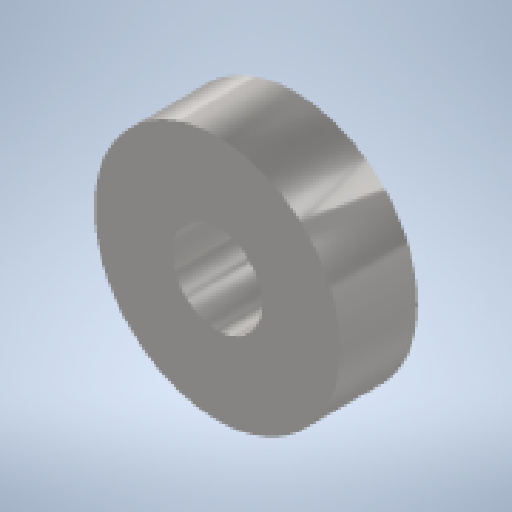
# Autodesk Inventor part: Metal bearing
Saved by Autodesk Inventor 2025.3 (Build 293356000, 356)
## iProperties
Created: 2025-08-19
Part Number: Metal bearing
Material: Stainless Steel
Document SubType Name: Modeling
Designer: sniel
Density: 8 g/cm^3
Appearance: Semi-Polished
Author: sniel
Autodesk Inventor part; units mm, degrees
ref_plane "YZ Plane" through (0, 0, 0) normal (1, 0, 0) x (0, 1, 0)
ref_plane "XZ Plane" through (0, 0, 0) normal (0, 1, 0) x (-1, 0, 0)
ref_plane "XY Plane" through (0, 0, 0) normal (0, 0, 1) x (1, 0, 0)
sketch "Sketch1" plane through (0, 0, 0) normal (0, 0, 1) x (1, 0, 0)
  circle A0 centre (32.4852, 19.5525) radius 11.1
  point P0 (0, 0)
  constraints: 1 centre point
extrude "Extrusion1" add sketch "Sketch1" along normal blind 7
sketch "Sketch7" plane through (32.4852, 19.5525, 7) normal (0, 0, 1) x (1, 0, 0)
  circle A0 centre (0, 0) radius 4.05
  circle A1 centre (0, 0) radius 11.1
  point P0 (-32.4852, -19.5525)
  constraints: 2 centre point
extrude "Extrusion7" cut sketch "Sketch7" against normal up to surface (7 mm away) contours A0
sketch "Sketch8" plane through (32.4852, 19.5525, 7) normal (0, 0, 1) x (1, 0, 0)
  circle A0 centre (0, 0) radius 4.05 projected
  line L0 (4.05, 0) -> (5.8, 0)
  circle A1 centre (0, 0) radius 5.8
  circle A2 centre (0, 0) radius 11.1 projected
  line L1 (11.1, 0) -> (9.35, 0)
  circle A3 centre (0, 0) radius 9.35
  point P0 (-32.4852, -19.5525)
  dimension "d18" = 1.75
  dimension "d19" = 1.75
  constraints: 4 end point, 4 horizontal alignment, 2 coincident, 2 horizontal, 6 other
  measures "d18" distance of L0.start L0.end
  measures "d19" distance of L1.start L1.end
extrude "Extrusion8" cut sketch "Sketch8" against normal blind 0.6 contours A3
sketch "Sketch9" plane through (32.4852, 19.5525, 0) normal (0, 0, -1) x (-1, 0, 0)
  circle A0 centre (0, 0) radius 5.8
  circle A1 centre (0, 0) radius 9.35
  point P0 (32.4852, -19.5525)
  constraints: 2 centre point
extrude "Extrusion9" cut sketch "Sketch9" against normal blind 0.6
body "Solid1"
